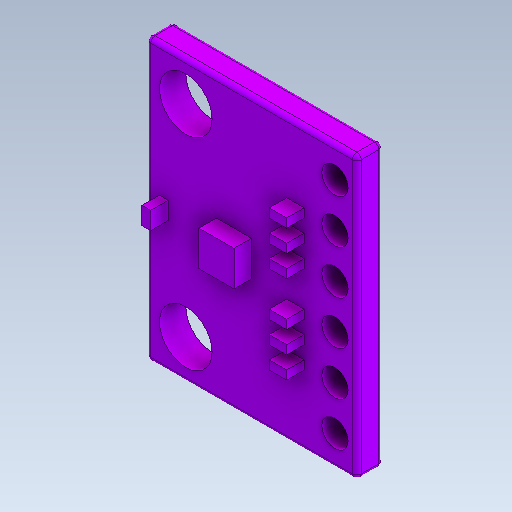
# Autodesk Inventor part: Czujnik BMP280
Saved by Autodesk Inventor 2020 (Build 240168000, 168)
## iProperties
Created: 2021-10-10
Part Number: Czujnik BMP280
Material: Ogólny
Document SubType Name: Modeling
Designer: Komputer
Density: 1 g/cm^3
Appearance: Domyślna
Mass: 0.256828 g
Surface Area: 5.05473 cm^2
Volume: 0.256828 cm^3
Author: Komputer
Autodesk Inventor part; units mm, degrees
ref_plane "YZ Plane" through (0, 0, 0) normal (1, 0, 0) x (0, 1, 0)
ref_plane "XZ Plane" through (0, 0, 0) normal (0, 1, 0) x (-1, 0, 0)
ref_plane "XY Plane" through (0, 0, 0) normal (0, 0, 1) x (1, 0, 0)
sketch "Szkic1" plane through (0, 0, 0) normal (0, 0, 1) x (1, 0, 0)
  point P0 (0, 0)
sketch "Szkic2" plane through (0, 0, 0) normal (0, 0, 1) x (1, 0, 0)
  line L0 (6, -8) -> (-6, -8)
  line L1 (-6, -8) -> (-6, 8)
  line L2 (-6, 8) -> (6, 8)
  line L3 (6, 8) -> (6, -8)
  line L4 (6, -8) -> (-6, 8) construction
  line L5 (-6, -8) -> (6, 8) construction
  point P0 (0, 0)
  dimension "d0" = 12
  dimension "d1" = 16
  constraints: 12 end point, 2 midpoint, 2 parallel, 1 horizontal, 1 perpendicular
  measures "d0" distance of L1.end L2.end
  measures "d1" distance of L0.end L1.end
extrude "Wyciągnięcie proste1" add sketch "Szkic2" along normal blind 1.5
fillet "Zaokrąglenie1" radius 0.25 12 edges at (0, 8, 1.5) (0, 8, 0) (6, 0, 1.5) (6, 0, 0) (0, -8, 1.5) (0, -8, 0) (6, -8, 0.75) (6, 8, 0.75) (-6, 0, 1.5) (-6, 0, 0) (-6, -8, 0.75) (-6, 8, 0.75)
sketch "Szkic3" plane through (0, 0, 1.5) normal (0, 0, 1) x (1, 0, 0)
  line L0 (-5.75, -7.75) -> (-5.75, 7.75) projected
  line L1 (-5.75, -7.75) -> (-3.75, -7.75)
  line L2 (5.75, -7.75) -> (-5.75, -7.75) projected
  line L3 (-3.75, -7.75) -> (-3.75, -5.75)
  line L4 (-5.75, 7.75) -> (5.75, 7.75) projected
  line L5 (-5.75, 7.75) -> (-3.75, 7.75)
  line L6 (-3.75, 7.75) -> (-3.75, 5.75)
  line L7 (5.75, 7.75) -> (4.75, 7.75)
  line L8 (4.75, 7.75) -> (4.75, 6.25)
  line L9 (4.75, 6.25) -> (4.75, 3.75)
  line L10 (4.75, 3.75) -> (4.75, 1.25)
  line L11 (4.75, 1.25) -> (4.75, -1.25)
  line L12 (4.75, -1.25) -> (4.75, -3.75)
  line L13 (4.75, -3.75) -> (4.75, -6.25)
  circle A0 centre (-3.75, 5.75) radius 1.5
  circle A1 centre (-3.75, -5.75) radius 1.5
  circle A2 centre (4.75, -6.25) radius 0.5
  circle A3 centre (4.75, -3.75) radius 0.75
  circle A4 centre (4.75, -6.25) radius 0.75
  circle A5 centre (4.75, -1.25) radius 0.75
  circle A6 centre (4.75, 1.25) radius 0.75
  circle A7 centre (4.75, 3.75) radius 0.75
  circle A8 centre (4.75, 6.25) radius 0.75
  point P0 (0, 0)
  dimension "d5" = 2
  dimension "d6" = 2
  dimension "d7" = 2
  dimension "d8" = 2
  dimension "d9" = 1
  dimension "d10" = 1.5
  dimension "d11" = 2.5
  dimension "d12" = 2.5
  dimension "d13" = 2.5
  dimension "d14" = 2.5
  dimension "d15" = 2.5
  dimension "d17" = 3
  dimension "d18" = 3
  dimension "d19" = 1
  dimension "d20" = 1.5
  dimension "d21" = 1.5
  dimension "d22" = 1.5
  dimension "d23" = 1.5
  dimension "d24" = 1.5
  dimension "d25" = 1.5
  constraints: 22 end point, 9 centre point, 9 coincident, 8 point on line, 3 perpendicular
  measures "d5" distance of L0.start L1.end
  measures "d6" distance of L1.end L3.end
  measures "d7" distance of L0.end L5.end
  measures "d8" distance of L5.end L6.end
  measures "d9" distance of L4.end L7.end
  measures "d10" distance of L7.end L8.end
  measures "d11" distance of L8.end L9.end
  measures "d12" distance of L9.end L10.end
  measures "d13" distance of L10.end L11.end
  measures "d14" distance of L11.end L12.end
  measures "d15" distance of L12.end L13.end
  measures "d17" diameter of A0
  measures "d18" diameter of A1
  measures "d19" diameter of A2
  measures "d20" diameter of A3
  measures "d21" diameter of A4
  measures "d22" diameter of A5
  measures "d23" diameter of A6
  measures "d24" diameter of A7
  measures "d25" diameter of A8
extrude "Wyciągnięcie proste2" cut sketch "Szkic3" against normal blind 1.5 contours A2 | A4 | A3 L13 L12 | L12 L13 A3 | A5 L12 L11 | L11 L12 A5 | A6 L11 L10 | L10 L11 A6 | A7 L10 L9 | L9 L10 A7 | A8 L9 L8 | L8 L9 A8 | A0 | A1
sketch "Szkic4" plane through (0, 0, 1.5) normal (0, 0, 1) x (1, 0, 0)
  line L0 (3, -3.5) -> (2, -3.5)
  line L1 (2, -3.5) -> (2, -4)
  line L2 (2, -4) -> (3, -4)
  line L3 (3, -4) -> (3, -3.5)
  line L4 (3, -3.5) -> (2, -4) construction
  line L5 (2, -3.5) -> (3, -4) construction
  line L6 (3, -2.25) -> (2, -2.25)
  line L7 (2, -2.25) -> (2, -2.75)
  line L8 (2, -2.75) -> (3, -2.75)
  line L9 (3, -2.75) -> (3, -2.25)
  line L10 (3, -2.25) -> (2, -2.75) construction
  line L11 (2, -2.25) -> (3, -2.75) construction
  line L12 (3, -1) -> (2, -1)
  line L13 (2, -1) -> (2, -1.5)
  line L14 (2, -1.5) -> (3, -1.5)
  line L15 (3, -1.5) -> (3, -1)
  line L16 (3, -1) -> (2, -1.5) construction
  line L17 (2, -1) -> (3, -1.5) construction
  line L18 (3, 1.5) -> (2, 1.5)
  line L19 (2, 1.5) -> (2, 1)
  line L20 (2, 1) -> (3, 1)
  line L21 (3, 1) -> (3, 1.5)
  line L22 (3, 1.5) -> (2, 1) construction
  line L23 (2, 1.5) -> (3, 1) construction
  line L24 (3, 2.75) -> (2, 2.75)
  line L25 (2, 2.75) -> (2, 2.25)
  line L26 (2, 2.25) -> (3, 2.25)
  line L27 (3, 2.25) -> (3, 2.75)
  line L28 (3, 2.75) -> (2, 2.25) construction
  line L29 (2, 2.75) -> (3, 2.25) construction
  line L30 (3, 4) -> (2, 4)
  line L31 (2, 4) -> (2, 3.5)
  line L32 (2, 3.5) -> (3, 3.5)
  line L33 (3, 3.5) -> (3, 4)
  line L34 (3, 4) -> (2, 3.5) construction
  line L35 (2, 4) -> (3, 3.5) construction
  line L36 (-2, -1) -> (0, -1)
  line L37 (0, -1) -> (0, 1)
  line L38 (0, 1) -> (-2, 1)
  line L39 (-2, 1) -> (-2, -1)
  line L40 (-2, -1) -> (0, 1) construction
  line L41 (0, -1) -> (-2, 1) construction
  line L42 (-4.75, -0.5) -> (-5.25, -0.5)
  line L43 (-5.25, -0.5) -> (-5.25, 0.5)
  line L44 (-5.25, 0.5) -> (-4.75, 0.5)
  line L45 (-4.75, 0.5) -> (-4.75, -0.5)
  line L46 (-4.75, -0.5) -> (-5.25, 0.5) construction
  line L47 (-5.25, -0.5) -> (-4.75, 0.5) construction
  point P0 (0, 0)
  point P1 (2.5, -3.75)
  point P2 (2.5, -2.5)
  point P3 (2.5, -1.25)
  point P4 (2.5, 1.25)
  point P5 (2.5, 2.5)
  point P6 (2.5, 3.75)
  point P7 (-1, 0)
  point P8 (-5, 0)
  dimension "d28" = 1
  dimension "d29" = 0.5
  dimension "d30" = 1
  constraints: 96 end point, 16 midpoint, 16 parallel, 8 horizontal, 8 perpendicular, 4 point on line
  measures "d28" distance of L2.end L1.end
  measures "d29" distance of L1.end L0.end
  measures "d30" distance of L42.end L43.end
extrude "Wyciągnięcie proste3" add sketch "Szkic4" along normal blind 1
